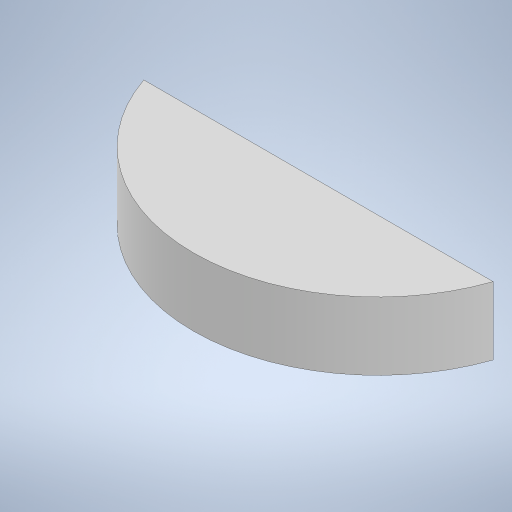
# Autodesk Inventor part: Tapa2
Saved by Autodesk Inventor 2024 (Build 280153000, 153)
## iProperties
Created: 2024-05-21
Part Number: Tapa2
Material: Genérico
Document SubType Name: Modeling
Designer: psepu
Density: 1 g/cm^3
Appearance: Valor por defecto
Author: psepu
Autodesk Inventor part; units mm, degrees
ref_plane "YZ Plane" through (0, 0, 0) normal (1, 0, 0) x (0, 1, 0)
ref_plane "XZ Plane" through (0, 0, 0) normal (0, 1, 0) x (-1, 0, 0)
ref_plane "XY Plane" through (0, 0, 0) normal (0, 0, 1) x (1, 0, 0)
sketch "Boceto1" plane through (0, 0, 0) normal (0, 0, 1) x (1, 0, 0)
  line L0 (0, 35) -> (0, 38)
  line L1 (0, 38) -> (-103.4, 38)
  line L2 (-103.4, 38) -> (-103.4, 0)
  line L3 (-103.4, 0) -> (-100.2, 0)
  line L4 (-100.2, 0) -> (-100.2, 35)
  line L5 (-100.2, 35) -> (-96.8, 35)
  line L6 (-96.8, 35) -> (-96.8, 0)
  line L7 (-96.8, 0) -> (-93.6, 0)
  line L8 (-93.6, 0) -> (-93.6, 35)
  line L9 (-93.6, 35) -> (0, 35)
  point P0 (0, 0)
  dimension "d0" = 38
  dimension "d1" = 103.4
  dimension "d2" = 3.2
  dimension "d3" = 35
  dimension "d4" = 3.4
  dimension "d5" = 3.2
  constraints: 20 end point, 6 perpendicular, 4 point on line, 1 horizontal, 1 vertical
  measures "d0" distance of point (0, 0) L0.end
  measures "d1" distance of L0.end L1.end
  measures "d2" distance of L2.end L3.end
  measures "d3" distance of L3.end L4.end
  measures "d4" distance of L4.end L5.end
  measures "d5" distance of L6.end L7.end
revolve "Revolución1" add sketch "Boceto1" angle 180 about axis through (0, 35, 0) along (0, 1, 0)
sketch "Boceto2" plane through (-103.4, 38, 0) normal (0, 1, 0) x (1, 0, 0)
  line L0 (103.4, 0) -> (103.4, -103.4)
  arc A0 (0, 0) -> (206.8, 0) centre (103.4, 0) ccw projected
  line L1 (103.4, -103.4) -> (103.4, -33.4)
  line L2 (103.4, -33.4) -> (201.257, -33.4)
  line L3 (103.4, -33.4) -> (5.543, -33.4)
  circle A1 centre (103.4, 0) radius 103.4
  line L4 (206.8, 0) -> (0, 0)
  dimension "d7" = 70
  constraints: 10 end point, 3 point on circle, 1 coincident, 1 horizontal, 1 perpendicular, 1 point on line, 1 vertical, 1 vertical alignment, 2 other
  measures "d7" distance of L0.end L1.end
extrude "Extrusión1" cut sketch "Boceto2" against normal blind 100 contours L4 A0 L2 L0 | L0 L3 A0 L4
